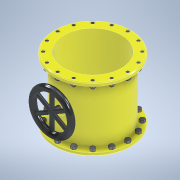
# Autodesk Inventor part: pipe_valve
Saved by Autodesk Inventor 2022 (Build 260153000, 153)
## iProperties
Created: 2021-12-16
Part Number: pipe_valve
Material: Steel
Document SubType Name: Modeling
Designer: jpc
Density: 7.85 g/cm^3
Appearance: Steel - Polished
Mass: 2.14484e+06 g
Surface Area: 119776 cm^2
Volume: 273228 cm^3
Author: jpc
Autodesk Inventor part; units mm, degrees
ref_plane "YZ Plane" through (0, 0, 0) normal (1, 0, 0) x (0, 1, 0)
ref_plane "XZ Plane" through (0, 0, 0) normal (0, 1, 0) x (-1, 0, 0)
ref_plane "XY Plane" through (0, 0, 0) normal (0, 0, 1) x (1, 0, 0)
sketch "cross_section" plane through (0, 0, 0) normal (0, 1, 0) x (-1, 0, 0)
  circle A0 centre (0, 0) radius 500
  circle A1 centre (0, 0) radius 450
  dimension "dia_out" = 1000
  dimension "dia_in" = 900
  constraints: 2 centre point, 2 coincident
  measures "dia_out" diameter of A0
  measures "dia_in" diameter of A1
sketch "curved_midline" plane through (0, 0, 0) normal (0, 0, 1) x (1, 0, 0)
  arc A0 (1000, 1000) -> (0, 0) centre (1000, 0) ccw
  line L0 (0, 0) -> (1000, 0) construction
  line L1 (1000, 0) -> (1000, 1000) construction
  dimension "d4" = 1000
  constraints: 4 end point, 2 point on circle, 1 centre point, 1 horizontal, 1 perpendicular
  measures "d4" distance of L0.end L1.end
sketch "straight_midline" plane through (0, 0, 0) normal (0, 0, 1) x (1, 0, 0)
  line L0 (0, 0) -> (0, 1000)
  dimension "len" = 1000
  constraints: 2 end point, 1 vertical
  measures "len" distance of L0.start L0.end
sweep "Sweep" add profiles "cross_section" path "straight_midline"
sketch "Sketch4" plane through (0, 0, 0) normal (0, -1, 0) x (1, 0, 0)
  circle A0 centre (0, 0) radius 600
  circle A1 centre (0, 0) radius 450 projected
  dimension "endcap_dia" = 1200
  constraints: 1 centre point, 1 coincident
  measures "endcap_dia" diameter of A0
extrude "Endcap" add sketch "Sketch4" against normal blind 50
ref_plane "Midplane" through (0, 500, 0) normal (0, -1, 0) x (1, 0, 0)
chamfer "Chamfer" distance 12.5 angle 45 1 edges at (-600, 0, 0)
sketch "Sketch7" plane through (0, 50, 0) normal (0, 1, 0) x (1, 0, 0)
  circle A0 centre (0, 0) radius 600 construction
  circle A1 centre (0, 0) radius 600 construction
  line L0 (-600, 0) -> (-499.1664, 0) construction
  circle A2 centre (-549.5832, 0) radius 25.2084
  circle A3 centre (0, 0) radius 450 projected
  circle A4 centre (0, 0) radius 500 projected
  dimension "d27" = 100.8336
  dimension "d28" = 50.4168
  constraints: 2 end point, 1 centre point, 1 horizontal, 1 horizontal alignment, 1 midpoint, 1 other
  measures "d27" distance of L0.start L0.end
  measures "d28" diameter of A2
extrude "Hole" cut sketch "Sketch7" against normal through all contours A2
pattern_circular "Holes" count 16 over 360 about axis through (0, -10, 0) along (0, 1, 0) of "Hole"
mirror "MirroredFeatures" about plane through (0, 500, 0) normal (0, -1, 0) of "Hole", "Holes", "Endcap", "Chamfer"
sketch "Sketch8" plane through (0, 50, 0) normal (0, 1, 0) x (1, 0, 0)
  circle A0 centre (-549.5832, 0) radius 25.2084 construction
  circle A1 centre (-549.5832, 0) radius 37.8126 construction
  circle A2 centre (0, 0) radius 587.5 construction
  line L0 (-587.5, 0) -> (-568.5416, 32.8369)
  line L1 (-568.5416, 32.8369) -> (-530.6248, 32.8369)
  line L2 (-530.6248, 32.8369) -> (-511.6664, 0)
  line L3 (-511.6664, 0) -> (-530.6248, -32.8369)
  line L4 (-530.6248, -32.8369) -> (-568.5416, -32.8369)
  line L5 (-568.5416, -32.8369) -> (-587.5, 0)
  dimension "d34" = 50.4168
  dimension "d35" = 75.6252
  constraints: 12 end point, 2 coincident, 1 centre point, 1 horizontal, 1 horizontal alignment, 14 other
  measures "d34" diameter of A0
  measures "d35" diameter of A1
extrude "BoltHead" add sketch "Sketch8" along normal blind 37.5 separate body
sketch "Sketch9" plane through (0, 50, 0) normal (0, -1, 0) x (1, 0, 0)
  circle A0 centre (-549.5832, 0) radius 25.2084 projected
  point P0 (0, 0)
extrude "BoltThreadHalf" add sketch "Sketch9" along normal blind 45 bodies 2
pattern_circular "BoltHalves" count 16 over 360 about axis through (0, -10, 0) along (0, 1, 0) bodies 2
mirror "MirroredBolts" about plane through (0, 500, 0) normal (0, -1, 0) bodies 2
sketch "Sketch10" plane through (-530.6248, 912.5, 32.8369) normal (0, -1, 0) x (0, 0, 1)
  circle A0 centre (-32.8369, 18.9584) radius 25.2084 projected
  point P0 (-32.8369, -530.6248)
extrude "ExtraThread" add sketch "Sketch10" along normal blind 22.5 bodies 2
chamfer "ThreadChamfer" distance 6.25 angle 45 1 edges at (-549.5832, 890, -25.2084)
pattern_circular "BoltNuts" count 16 over 360 about axis through (0, 950, 0) along (0, 1, 0) of "ExtraThread", "ThreadChamfer" bodies 2
sketch "Sketch12" plane through (0, 0, 0) normal (1, 0, 0) x (0, 1, 0)
  line L0 (50, 500) -> (950, 500) construction
  line L1 (12.5, 600) -> (50, 600) construction
  line L2 (0, 524.3748) -> (0, 574.7916) construction
  line L3 (50, 574.7916) -> (50, 524.3748) construction
  line L4 (1000, 450) -> (0, 450) construction
  line L5 (500, 450) -> (600, 450)
  line L6 (600, 450) -> (600, 524.3748)
  line L7 (600, 524.3748) -> (500, 524.3748)
  line L8 (500, 524.3748) -> (500, 450)
  line L9 (50, 524.3748) -> (0, 524.3748) projected
  point P0 (0, 0)
  dimension "d54" = 50
  dimension "d57" = 100
  constraints: 8 end point, 2 parallel, 1 collinear, 1 horizontal, 1 midpoint, 1 perpendicular
  measures "d54" distance between parallel lines of L2 L3
  measures "d57" distance of L6.end L7.end
revolve "ValveSleeve" add sketch "Sketch12" angle 360 about axis through (0, 500, 524.3748) along (0, 0, -1) bodies 1
sketch "Sketch13" plane through (0, 0, 0) normal (1, 0, 0) x (0, 1, 0)
  line L0 (950, 600) -> (987.5, 600) projected
  line L1 (1000, 450) -> (0, 450) projected
  line L2 (500, 450) -> (537.5, 450)
  line L3 (537.5, 450) -> (537.5, 637.5)
  line L4 (537.5, 637.5) -> (500, 637.5)
  line L5 (500, 637.5) -> (500, 450)
  line L6 (0, 524.3748) -> (0, 574.7916) projected
  line L7 (50, 574.7916) -> (50, 524.3748) projected
  point P0 (0, 0)
  dimension "d59" = 50
  dimension "d60" = 37.5
  dimension "d67" = 187.5
  dimension "d68" = 150
  constraints: 8 end point, 2 parallel, 1 horizontal, 1 midpoint, 1 perpendicular
  measures "d59" distance between parallel lines of L6 L7
  measures "d60" distance between parallel lines of L3 L5
  measures "d67" distance of L2.end L3.end
  measures "d68" distance between parallel lines of L0 L1
revolve "ValveAxis" add sketch "Sketch13" angle 360 about axis through (0, 500, 637.5) along (0, 0, -1) separate body
sketch "Sketch14" plane through (0, 0, 0) normal (1, 0, 0) x (0, 1, 0)
  line L0 (462.5, 637.5) -> (537.5, 637.5) construction
  arc A0 (500, 600) -> (500, 675) centre (500, 637.5) ccw
  circle A1 centre (800, 637.5) radius 46.875
  line L1 (500, 675) -> (500, 600)
  line L2 (800, 637.5) -> (500, 637.5) construction
  line L3 (400, 524.3748) -> (600, 524.3748) construction
  point P0 (0, 0)
  dimension "d62" = 200
  dimension "d63" = 300
  dimension "d64" = 75
  dimension "d65" = 93.75
  constraints: 5 end point, 3 point on circle, 2 centre point, 2 midpoint, 1 collinear, 1 vertical
  measures "d62" distance of L3.start L3.end
  measures "d63" distance of L2.start L2.end
  measures "d64" distance of L1.start L1.end
  measures "d65" diameter of A1
revolve "ValveHandle" add sketch "Sketch14" angle 360 about axis through (0, 500, 675) along (0, 0, -1) bodies 3
sketch "Sketch15" plane through (0, 0, 0) normal (1, 0, 0) x (0, 1, 0)
  line L0 (500, 609.375) -> (800, 609.375)
  line L1 (800, 609.375) -> (800, 637.5)
  line L2 (800, 637.5) -> (500, 637.5)
  line L3 (500, 637.5) -> (500, 609.375)
  arc A0 (537.5, 637.5) -> (462.5, 637.5) centre (500, 637.5) ccw projected
  arc A1 (800, 684.375) -> (800, 590.625) centre (800, 637.5) ccw projected
  line L4 (462.5, 637.5) -> (537.5, 637.5) projected
  line L5 (462.5, 450) -> (537.5, 450) projected
  point P0 (0, 0)
  dimension "d69" = 37.5
  dimension "d70" = 28.125
  constraints: 8 end point, 2 coincident, 2 parallel, 1 horizontal, 1 perpendicular
  measures "d69" radius of A0
  measures "d70" distance between parallel lines of L0 L2
revolve "ValveSpoke" add sketch "Sketch15" angle 360 about axis through (0, 800, 637.5) along (0, -1, 0) bodies 3 contours L3 L2 A1 L0 | A1 L2 L1 L0
pattern_circular "ValveSpokes" count 6 over 360 about axis through (0, 500, 543.75) along (0, 0, -1) of "ValveSpoke" bodies 3
equation "\"d4\" = dia_out"
equation "\"endcap_dia\" = 1.2 * dia_out"
equation "\"endcap_thick\" = -0.5 * dia_in + 0.5 * dia_out"
equation "\"d28\" = 0.5 * d27"
equation "\"d35\" = 1.5 * d34"
equation "\"bolt_thick\" = 0.75 * endcap_thick"
equation "\"d38\" = 0.9 * endcap_thick"
equation "\"d43\" = 0.45 * endcap_thick"
equation "\"d48\" = 0.125 * endcap_thick"
equation "\"d57\" = 2 * d54"
equation "\"d60\" = 0.75 * d59"
equation "\"d67\" = 1.25 * d68"
equation "\"d63\" = 1.5 * d62"
equation "\"d65\" = 1.25 * d64"
equation "\"d70\" = 0.75 * d69"
equation "\"d24\" = 0.25 * endcap_thick"
